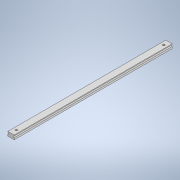
# Autodesk Inventor part: 滑轨
Saved by Autodesk Inventor 2020 (Build 240168000, 168)
## iProperties
Created: 2020-12-02
Part Number: 滑轨
Material: 常规
Document SubType Name: Sheet Metal
Designer: huang
Density: 1 g/cm^3
Sheet Metal Rule: 默认_mm
Appearance: 默认
Author: huang
Autodesk Inventor part; units mm, degrees
ref_plane "YZ Plane" through (0, 0, 0) normal (1, 0, 0) x (0, 1, 0)
ref_plane "XZ Plane" through (0, 0, 0) normal (0, 1, 0) x (-1, 0, 0)
ref_plane "XY Plane" through (0, 0, 0) normal (0, 0, 1) x (1, 0, 0)
sketch "草图1" plane through (0, 0, 0) normal (0, 1, 0) x (-1, 0, 0)
  line L0 (0, 0) -> (12, 0)
  line L1 (12, 0) -> (12, -300)
  line L2 (12, -300) -> (0, -300)
  line L3 (0, -300) -> (0, 0)
  dimension "d0" = 12
  dimension "d1" = 300
  constraints: 8 end point, 2 parallel, 1 horizontal, 1 perpendicular
  measures "d0" distance of L1.end L2.end
  measures "d1" distance of L0.end L1.end
extrude "拉伸1" add sketch "草图1" along normal blind 8
sketch "草图2" plane through (-12, 0, 0) normal (0, 0, 1) x (1, 0, 0)
  line L0 (0, 8) -> (0, 5)
  line L1 (0, 0) -> (0, 8) projected
  circle A0 centre (0, 5) radius 1.5
  line L2 (12, 8) -> (0, 8) projected
  line L3 (6, 8) -> (6, -1.6041)
  line L4 (12, 8) -> (12, 5)
  line L5 (12, 0) -> (12, 8)
  circle A1 centre (12, 5) radius 1.5
  line L6 (0, 8) -> (12, 8)
  point P0 (12, 6.5)
  point P1 (12, 3.5)
  point P2 (0, 6.5)
  point P3 (0, 3.5)
  dimension "d9" = 3
  dimension "d10" = 3
  constraints: 10 end point, 5 symmetric about line, 2 centre point, 2 coincident, 2 point on line, 1 midpoint, 1 vertical, 1 other
  measures "d9" distance of L0.start L0.end
  measures "d10" diameter of A0
extrude "拉伸2" cut sketch "草图2" against normal through all contours A0 L1 L0 | L4 L5 A1 picked at (0.7027, 4.2973) picked at (11.121, 5.4613)
sketch "草图3" plane through (0, 8, 0) normal (0, 1, 0) x (1, 0, 0)
  line L0 (-12, 0) -> (0, 0) projected
  line L1 (-6, 0) -> (-6, 10)
  circle A0 centre (-6, 10) radius 2
  line L2 (0, 300) -> (-12, 300) projected
  line L3 (-6, 300) -> (-6, 290)
  circle A1 centre (-6, 290) radius 2
  dimension "d11" = 10
  dimension "d12" = 4
  dimension "d13" = 10
  dimension "d14" = 4
  constraints: 4 end point, 2 centre point, 2 coincident, 2 midpoint, 2 vertical
  measures "d11" distance of L1.start L1.end
  measures "d12" diameter of A0
  measures "d13" distance of L3.start L3.end
  measures "d14" diameter of A1
extrude "拉伸3" cut sketch "草图3" against normal through all
equation "\"折弯半径\" = 厚度"
equation "\"折弯释压宽度\" = 厚度"
equation "\"折弯释压深度\" = 0.5 * 厚度"
equation "\"拐角释压尺寸\" = 4 * 厚度"
equation "\"最小余量\" = 2 * 厚度"
equation "\"过渡半径\" = 折弯半径"
equation "\"Jacobi半径尺寸\" = 折弯半径"
equation "\"间隙大小\" = 厚度"
equation "\"厚度\" = 0.5"
